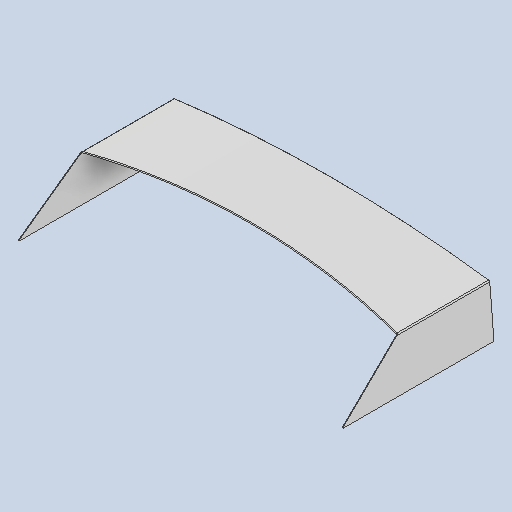
# Autodesk Inventor part: МОО 034 лист спина-холка
Saved by Autodesk Inventor 2024.2 (Build 282272000, 272)
## iProperties
Created: 2024-04-18
Part Number: МОО 034 лист спина-холка
Material: Stainless Steel AISI 304
Document SubType Name: Sheet Metal
Designer: admin
Stock Number: МОО 034 лист спина-холка
Density: 8 g/cm^3
Flat Pattern Width: 71.5519 cm
Flat Pattern Length: 197.5 cm
Flat Pattern Area: 14131.5 cm^2
Sheet Metal Rule: Default_mm
Sheet Metal Width: 715,519 mm
Sheet Metal Length: 1975,003 mm
Sheet Metal Area: 1413152,610 mm^2
Appearance: Default
Mass: 34137.4 g
Surface Area: 28609.5 cm^2
Volume: 4267.17 cm^3
Author: admin
Autodesk Inventor part; units mm, degrees
ref_plane "YZ Plane" through (0, 0, 0) normal (1, 0, 0) x (0, 1, 0)
ref_plane "XZ Plane" through (0, 0, 0) normal (0, 1, 0) x (-1, 0, 0)
ref_plane "XY Plane" through (0, 0, 0) normal (0, 0, 1) x (1, 0, 0)
sketch "Sketch1" plane through (0, 0, 0) normal (0, 0, 1) x (1, 0, 0)
  line L0 (-750, 0) -> (750, 0) construction
  line L1 (750, 0) -> (750, -2700) construction
  line L2 (750, -2700) -> (-750, -2700) construction
  line L3 (-750, -2700) -> (-750, 0) construction
  line L4 (800, 50) -> (-800, 50) construction
  line L5 (-800, 50) -> (-800, -2750) construction
  line L6 (-800, -2750) -> (800, -2750) construction
  line L7 (800, -2750) -> (800, 50) construction
  line L8 (-850, 100) -> (850, 100) construction
  line L9 (850, 100) -> (850, -2800) construction
  line L10 (850, -2800) -> (-850, -2800) construction
  line L11 (-850, -2800) -> (-850, 100) construction
  arc A0 (750, 0) -> (745.2706, 0.6314) centre (0, -5600) ccw construction
  line L12 (-750, -2100) -> (750, -2100) construction
  line L13 (114.1118, -2698.3696) -> (750, -2100) construction
  arc A1 (750, -2100) -> (770.156, -238.4205) centre (-10250, -1050) ccw construction
  line L14 (750, 0) -> (749.6018, -2.9735) construction
  arc A2 (750, -3.0268) -> (0, 47) centre (-0.2, -5603) ccw construction
  line L15 (750, 0) -> (747.0136, -0.2851) construction
  arc A3 (767.1641, -238.6409) -> (747.4657, -5.0326) centre (-10252.9895, -1050.2527) ccw construction
  arc A4 (750.4522, -4.7486) -> (745.2706, 0.6314) centre (744.4791, -5.3162) ccw
  arc A5 (747.4657, -5.0326) -> (744.8748, -2.3426) centre (744.4792, -5.3164) ccw construction
  line L16 (750, -2100) -> (752.9864, -2100.2851) construction
  arc A6 (752.9864, -2100.2851) -> (771.2831, -213.263) centre (-10246.9891, -1050.0292) ccw construction
  line L17 (750, -2100) -> (752.0559, -2102.1848) construction
  line L18 (752.0559, -2102.1848) -> (752.0559, -2102.1848) construction
  arc A7 (749.1768, -2100.7746) -> (750.1074, -2098.8746) centre (747.1209, -2098.5898) ccw construction
  line L19 (0, -2697) -> (110, -2697) construction
  line L20 (112.0559, -2696.1848) -> (685.3133, -2156.7506) construction
  arc A8 (110, -2700) -> (114.1118, -2698.3696) centre (110, -2694) ccw construction
  arc A9 (110, -2697) -> (112.0559, -2696.1848) centre (110, -2694) ccw construction
  line L21 (685.3133, -2156.7506) -> (687.3692, -2158.9354) construction
  line L22 (752.0559, -2102.1848) -> (671.2185, -2178.2526) construction
  line L23 (671.2185, -2178.2526) -> (669.1626, -2176.0678) construction
  arc A10 (747.4657, -5.0326) -> (747.0136, -0.2851) centre (-10252.9895, -1050.2527) ccw construction
  arc A11 (745.2706, 0.6314) -> (0, 50) centre (0, -5600) ccw
  arc A12 (750.4522, -4.7486) -> (750, 0) centre (-10250, -1050) ccw construction
  line L24 (770.156, -238.4205) -> (767.1641, -238.6409) construction
  line L25 (768.2917, -213.4901) -> (771.2831, -213.263) construction
  arc A13 (770.156, -238.4205) -> (750.4522, -4.7486) centre (-10250, -1050) ccw
  line L26 (0, 100) -> (0, 50) construction
  line L27 (0, -2700) -> (0, -2697) construction
  line L28 (0, 47) -> (0, 0) construction
  line L29 (0, 50) -> (0, 47) construction
  arc A14 (752.0559, -2102.1848) -> (752.9864, -2100.2851) centre (749.9998, -2099.9999) ccw construction
  point P0 (0, -2750)
  dimension "d54" = 1500
  dimension "d55" = 2700
  dimension "d58" = 2100
  dimension "d68" = 6
  dimension "d70" = 3
  dimension "d75" = 3
  dimension "d83" = 6
  dimension "d86" = 3
  dimension "d112" = 239.271
  dimension "d113" = 50
  dimension "d114" = 50
  dimension "d115" = 3
  dimension "d117" = 110
  dimension "d118" = 25
  dimension "d119" = 111
  dimension "d120" = 25
  measures "d54" distance of L0.start L0.end
  measures "d55" distance of L0.end L1.end
  measures "d58" distance between parallel lines of L12 L0
  measures "d68" radius of A4
  measures "d70" radius of A5
  measures "d75" radius of A7
  measures "d83" radius of A8
  measures "d86" radius of A9
  measures "d112" distance of L24.start L0.end
  measures "d113" distance between parallel lines of L4 L8
  measures "d114" distance between parallel lines of L0 L4
  measures "d115" distance of L26.end L28.start
  measures "d117" distance from line of L27 A8.centre
  measures "d118" distance of L23.end L21.end
  measures "d119" distance of L12.end L23.end
  measures "d120" distance of L24.start L25.start
contour flange "Contour Flange2" sketch "Sketch1" thickness 3 bend radius 3 width 720 along (0, 0, 1) mid plane no both sides no wall seen from (760.924, -121.5323, 0) lies toward (-0.9964637, -0.0840242, 0) curves A13 A4 A11
bend "Bend2"
corner "Corner2"
mirror "Mirror2" about plane through (0, 0, 0) normal (1, 0, 0) of "Contour Flange2"
sketch "Sketch2" plane through (0, 0, 0) normal (1, 0, 0) x (0, 1, 0)
  line L0 (50, 720) -> (-238.6409, 720)
  line L1 (50, 375.0112) -> (50, 720)
  line L2 (50, 375.0112) -> (-238.6409, 719)
  line L3 (-238.6409, 720) -> (-238.6409, 0) projected
  point P0 (0, 0)
  dimension "d127" = 1
  dimension "d129" = 40
  constraints: 6 end point, 1 perpendicular, 1 point on line
  measures "d127" distance of L0.end L2.end
  measures "d129" angle of L3 L2
extrude "Extrusion2" cut sketch "Sketch2" along normal through all both and the other way through all
fillet "Fillet1" radius 2 2 edges at (-768.6601, -238.5307, 718.8687) (768.6601, -238.5307, 718.8687)
equation "\"d36\" = Thickness"
equation "\"d37\" = BendReliefWidth"
equation "\"d38\" = BendReliefDepth"
equation "\"d39\" = MinimumRemnant"
equation "\"d40\" = TransitionRadius"
equation "\"d42\" = BendRadius"
equation "\"d44\" = CornerReliefSize"
equation "\"d45\" = GapSize"
equation "\"d46\" = JacobiRadiusSize"
equation "\"BendRadius\" = Thickness"
equation "\"BendReliefWidth\" = Thickness"
equation "\"BendReliefDepth\" = 0.5 * Thickness"
equation "\"CornerReliefSize\" = 4 * Thickness"
equation "\"MinimumRemnant\" = 2 * Thickness"
equation "\"TransitionRadius\" = BendRadius"
equation "\"JacobiRadiusSize\" = BendRadius"
equation "\"GapSize\" = Thickness"
equation "\"Thickness\" = 3"
body "Solid3"
